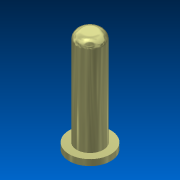
# Autodesk Inventor part: 2.1mm DC Power Socket Pin
Saved by Autodesk Inventor 2013 (Build 170138000, 138)
## iProperties
Created: 2012-05-07
Material: Copper
Document SubType Name: Modeling
Designer: sdarley
Density: 1 g/cm^3
Project: 2.1mm DC Power Socket
Description: 2.1mm DC Power Socket Pin
Author: sdarley
Title: 2.1mm DC Power Socket Pin
Revision Number: 1
Autodesk Inventor part; units mm, degrees
ref_plane "YZ Plane" through (0, 0, 0) normal (1, 0, 0) x (0, 1, 0)
ref_plane "XZ Plane" through (0, 0, 0) normal (0, 1, 0) x (-1, 0, 0)
ref_plane "XY Plane" through (0, 0, 0) normal (0, 0, 1) x (1, 0, 0)
sketch "Sketch1" plane through (0, 0, 0) normal (0, 0, 1) x (1, 0, 0)
  circle A0 centre (0, 0) radius 1.725
  dimension "d0" = 3.45
  constraints: 1 centre point, 1 coincident
  measures "d0" diameter of A0
extrude "Extrusion1" add sketch "Sketch1" along normal blind 0.5
sketch "Sketch2" plane through (0, 0, 0.5) normal (0, 0, 1) x (1, 0, 0)
  circle A0 centre (0, 0) radius 1.725 projected
  circle A1 centre (0, 0) radius 1.1
  dimension "d3" = 2.2
  constraints: 1 centre point, 1 coincident
  measures "d3" diameter of A1
extrude "Extrusion2" add sketch "Sketch2" along normal blind 8 contours A1
fillet "Fillet1" radius 0.6 1 edges at (-1.1, 0, 8.5)
body "Solid1"
